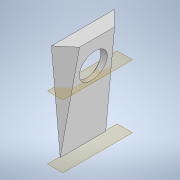
# Autodesk Inventor part: irragation01
Saved by Autodesk Inventor 2021 (Build 250183000, 183)
## iProperties
Created: 2020-07-06
Part Number: irragation01
Material: Generic
Document SubType Name: Modeling
Designer: robst
Density: 1 g/cm^3
Appearance: Default
Author: robst
Autodesk Inventor part; units mm, degrees
ref_plane "YZ Plane" through (0, 0, 0) normal (1, 0, 0) x (0, 1, 0)
ref_plane "XY Plane" through (0, 0, 0) normal (0, 0, 1) x (1, 0, 0)
sketch "Sketch1" plane through (0, 0, 0) normal (0, 0, 1) x (1, 0, 0)
  line L0 (0, 0) -> (14.2789, 101.6)
  line L1 (14.2789, 101.6) -> (0, 101.6)
  line L2 (0, 101.6) -> (0, 0)
  dimension "height" = 101.6
  dimension "d1" = 8
  dimension "d2" = 14.279
  constraints: 6 end point, 1 horizontal, 1 vertical
  measures "height" distance from line of L0.start L1
  measures "d1" angle of L0 L2
  measures "d2" distance of L0.end L1.end
extrude "MainStructure" add sketch "Sketch1" along normal mid plane 63.5
sketch "Sketch2" plane through (0, 0, 31.75) normal (-1, 0, 0) x (0, 0, 1)
  circle A0 centre (-31.75, 73.66) radius 13.97
  line L0 (-63.5, 101.6) -> (0, 101.6) projected
  line L1 (-31.75, 101.6) -> (-31.75, 0) construction
  dimension "hole" = 27.94
  dimension "centerOfHoleFromTop" = 27.94
  dimension "d29" = 0
  constraints: 2 end point, 1 centre point, 1 midpoint, 1 vertical
  measures "hole" diameter of A0
  measures "centerOfHoleFromTop" distance from line of A0.centre L0
  measures "d29" distance from line of A0.centre L1
extrude "PipeHole" cut sketch "Sketch2" against normal through all
sketch "Sketch6" plane through (0, 0, 0) normal (0, 0, 1) x (1, 0, 0)
  line L0 (0, 101.6) -> (14.2789, 101.6) projected
  line L1 (0, 0) -> (0, 101.6) projected
  line L2 (14.2789, 101.6) -> (0, 0) projected
  line L3 (0, 101.6) -> (14.1055, 100.3659)
  line L4 (14.1055, 100.3659) -> (14.2789, 101.6)
  line L5 (14.2789, 101.6) -> (0, 101.6)
  dimension "mainAngle" = 5
  constraints: 6 end point, 1 collinear, 1 point on line
  measures "mainAngle" angle of L3 L0
extrude "AngleForTopRelief" cut sketch "Sketch6" along normal through all both and the other way through all contours L0 L2 L3
sketch "Sketch7" plane through (0, 0, -31.75) normal (-1, 0, 0) x (0, 0, 1)
  line L0 (0, 0) -> (0, 101.6) construction
  line L1 (0, 44.45) -> (63.5, 44.45) construction
  line L2 (63.5, 0) -> (63.5, 100.3659) construction
  line L3 (0, 0) -> (63.5, 0) projected
  line L4 (9.9151, 38.1) -> (7.9473, 38.1)
  line L5 (7.9473, 38.1) -> (7.9473, 38.6187)
  line L6 (7.9473, 38.6187) -> (8.5936, 38.6187)
  line L7 (8.5936, 38.6187) -> (8.5936, 42.6613)
  line L8 (8.5936, 42.6613) -> (7.9473, 42.6613)
  line L9 (7.9473, 42.6613) -> (7.9473, 43.18)
  line L10 (7.9473, 43.18) -> (9.9151, 43.18)
  line L11 (9.9151, 43.18) -> (9.9151, 42.6613)
  line L12 (9.9151, 42.6613) -> (9.2687, 42.6613)
  line L13 (9.2687, 42.6613) -> (9.2687, 38.6187)
  line L14 (9.2687, 38.6187) -> (9.9151, 38.6187)
  line L15 (9.9151, 38.6187) -> (9.9151, 38.1)
  line L16 (14.6822, 38.1) -> (13.8053, 38.1)
  line L17 (13.8053, 38.1) -> (12.1998, 40.1213)
  line L18 (12.1998, 40.1213) -> (11.4259, 40.1213)
  line L19 (11.4259, 40.1213) -> (11.4259, 38.1)
  line L20 (11.4259, 38.1) -> (10.7507, 38.1)
  line L21 (10.7507, 38.1) -> (10.7507, 43.18)
  line L22 (10.7507, 43.18) -> (12.0599, 43.18)
  spline S0 degree 2 poles (12.0599, 43.18) (12.4962, 43.18) (13.0849, 43.0853) (13.3525, 42.9124) knots 0 0 0 1 2 2 2
  spline S1 degree 2 poles (13.3525, 42.9124) (13.6201, 42.7395) (13.9288, 42.2002) (13.9288, 41.8009) knots 0 0 0 1 2 2 2
  spline S2 degree 2 poles (13.9288, 41.8009) (13.9288, 41.2452) (13.3607, 40.4918) (12.875, 40.3107) knots 0 0 0 1 2 2 2
  line L23 (12.875, 40.3107) -> (14.6822, 38.1)
  spline S3 degree 2 poles (13.2249, 41.7474) (13.2249, 41.9697) (13.0684, 42.3114) (12.9038, 42.4225) knots 0 0 0 1 2 2 2
  spline S4 degree 2 poles (12.9038, 42.4225) (12.7597, 42.5172) (12.3768, 42.5954) (12.0969, 42.5954) knots 0 0 0 1 2 2 2
  line L24 (12.0969, 42.5954) -> (11.4259, 42.5954)
  line L25 (11.4259, 42.5954) -> (11.4259, 40.6853)
  line L26 (11.4259, 40.6853) -> (12.0187, 40.6853)
  spline S5 degree 2 poles (12.0187, 40.6853) (12.311, 40.6853) (12.7762, 40.7882) (12.9367, 40.9488) knots 0 0 0 1 2 2 2
  spline S6 degree 2 poles (12.9367, 40.9488) (13.0849, 41.0887) (13.2249, 41.4839) (13.2249, 41.7474) knots 0 0 0 1 2 2 2
  line L27 (19.0171, 38.1) -> (18.1402, 38.1)
  line L28 (18.1402, 38.1) -> (16.5347, 40.1213)
  line L29 (16.5347, 40.1213) -> (15.7608, 40.1213)
  line L30 (15.7608, 40.1213) -> (15.7608, 38.1)
  line L31 (15.7608, 38.1) -> (15.0856, 38.1)
  line L32 (15.0856, 38.1) -> (15.0856, 43.18)
  line L33 (15.0856, 43.18) -> (16.3947, 43.18)
  spline S7 degree 2 poles (16.3947, 43.18) (16.8311, 43.18) (17.4198, 43.0853) (17.6874, 42.9124) knots 0 0 0 1 2 2 2
  spline S8 degree 2 poles (17.6874, 42.9124) (17.955, 42.7395) (18.2637, 42.2002) (18.2637, 41.8009) knots 0 0 0 1 2 2 2
  spline S9 degree 2 poles (18.2637, 41.8009) (18.2637, 41.2452) (17.6956, 40.4918) (17.2098, 40.3107) knots 0 0 0 1 2 2 2
  line L34 (17.2098, 40.3107) -> (19.0171, 38.1)
  spline S10 degree 2 poles (17.5598, 41.7474) (17.5598, 41.9697) (17.4033, 42.3114) (17.2387, 42.4225) knots 0 0 0 1 2 2 2
  spline S11 degree 2 poles (17.2387, 42.4225) (17.0946, 42.5172) (16.7117, 42.5954) (16.4318, 42.5954) knots 0 0 0 1 2 2 2
  line L35 (16.4318, 42.5954) -> (15.7608, 42.5954)
  line L36 (15.7608, 42.5954) -> (15.7608, 40.6853)
  line L37 (15.7608, 40.6853) -> (16.3536, 40.6853)
  spline S12 degree 2 poles (16.3536, 40.6853) (16.6459, 40.6853) (17.111, 40.7882) (17.2716, 40.9488) knots 0 0 0 1 2 2 2
  spline S13 degree 2 poles (17.2716, 40.9488) (17.4198, 41.0887) (17.5598, 41.4839) (17.5598, 41.7474) knots 0 0 0 1 2 2 2
  line L38 (18.873, 38.1) -> (20.5855, 43.18)
  line L39 (20.5855, 43.18) -> (21.4171, 43.18)
  line L40 (21.4171, 43.18) -> (23.1296, 38.1)
  line L41 (23.1296, 38.1) -> (22.4175, 38.1)
  line L42 (22.4175, 38.1) -> (21.9564, 39.5203)
  line L43 (21.9564, 39.5203) -> (20.0174, 39.5203)
  line L44 (20.0174, 39.5203) -> (19.5564, 38.1)
  line L45 (19.5564, 38.1) -> (18.873, 38.1)
  line L46 (21.7711, 40.0966) -> (20.9848, 42.4884)
  line L47 (20.9848, 42.4884) -> (20.2027, 40.0966)
  line L48 (20.2027, 40.0966) -> (21.7711, 40.0966)
  spline S14 degree 2 poles (25.8055, 38.0012) (25.2662, 38.0012) (24.3729, 38.3305) (24.0518, 38.664) knots 0 0 0 1 2 2 2
  spline S15 degree 2 poles (24.0518, 38.664) (23.7307, 39.0016) (23.389, 39.9978) (23.389, 40.6441) knots 0 0 0 1 2 2 2
  spline S16 degree 2 poles (23.389, 40.6441) (23.389, 41.2575) (23.7348, 42.229) (24.0559, 42.5748) knots 0 0 0 1 2 2 2
  spline S17 degree 2 poles (24.0559, 42.5748) (24.3647, 42.9083) (25.2703, 43.2706) (25.8096, 43.2706) knots 0 0 0 1 2 2 2
  spline S18 degree 2 poles (25.8096, 43.2706) (26.069, 43.2706) (26.5383, 43.1965) (26.7523, 43.1306) knots 0 0 0 1 2 2 2
  spline S19 degree 2 poles (26.7523, 43.1306) (26.9252, 43.0812) (27.3451, 42.9001) (27.4728, 42.8342) knots 0 0 0 1 2 2 2
  line L49 (27.4728, 42.8342) -> (27.4728, 42.0191)
  line L50 (27.4728, 42.0191) -> (27.4151, 42.0191)
  spline S20 degree 2 poles (27.4151, 42.0191) (27.2875, 42.1302) (27.0199, 42.332) (26.7729, 42.4472) knots 0 0 0 1 2 2 2
  spline S21 degree 2 poles (26.7729, 42.4472) (26.5671, 42.5501) (26.036, 42.686) (25.7314, 42.686) knots 0 0 0 1 2 2 2
  spline S22 degree 2 poles (25.7314, 42.686) (24.9986, 42.686) (24.0929, 41.5827) (24.0929, 40.6647) knots 0 0 0 1 2 2 2
  spline S23 degree 2 poles (24.0929, 40.6647) (24.0929, 40.1542) (24.3317, 39.3885) (24.5581, 39.1251) knots 0 0 0 1 2 2 2
  spline S24 degree 2 poles (24.5581, 39.1251) (24.7763, 38.8616) (25.3938, 38.5858) (25.7808, 38.5858) knots 0 0 0 1 2 2 2
  spline S25 degree 2 poles (25.7808, 38.5858) (26.0648, 38.5858) (26.6329, 38.6681) (26.8264, 38.7504) knots 0 0 0 1 2 2 2
  line L51 (26.8264, 38.7504) -> (26.8264, 40.0637)
  line L52 (26.8264, 40.0637) -> (25.6491, 40.0637)
  line L53 (25.6491, 40.0637) -> (25.6491, 40.6565)
  line L54 (25.6491, 40.6565) -> (27.4933, 40.6565)
  line L55 (27.4933, 40.6565) -> (27.4933, 38.4376)
  spline S26 degree 2 poles (27.4933, 38.4376) (27.3657, 38.3799) (26.9294, 38.2029) (26.7441, 38.1494) knots 0 0 0 1 2 2 2
  spline S27 degree 2 poles (26.7441, 38.1494) (26.493, 38.0753) (26.0895, 38.0012) (25.8055, 38.0012) knots 0 0 0 1 2 2 2
  line L56 (27.7939, 38.1) -> (29.5064, 43.18)
  line L57 (29.5064, 43.18) -> (30.338, 43.18)
  line L58 (30.338, 43.18) -> (32.0505, 38.1)
  line L59 (32.0505, 38.1) -> (31.3383, 38.1)
  line L60 (31.3383, 38.1) -> (30.8773, 39.5203)
  line L61 (30.8773, 39.5203) -> (28.9383, 39.5203)
  line L62 (28.9383, 39.5203) -> (28.4772, 38.1)
  line L63 (28.4772, 38.1) -> (27.7939, 38.1)
  line L64 (30.692, 40.0966) -> (29.9057, 42.4884)
  line L65 (29.9057, 42.4884) -> (29.1235, 40.0966)
  line L66 (29.1235, 40.0966) -> (30.692, 40.0966)
  line L67 (33.7836, 38.1) -> (33.7836, 42.579)
  line L68 (33.7836, 42.579) -> (32.0793, 42.579)
  line L69 (32.0793, 42.579) -> (32.0793, 43.18)
  line L70 (32.0793, 43.18) -> (36.1631, 43.18)
  line L71 (36.1631, 43.18) -> (36.1631, 42.579)
  line L72 (36.1631, 42.579) -> (34.4588, 42.579)
  line L73 (34.4588, 42.579) -> (34.4588, 38.1)
  line L74 (34.4588, 38.1) -> (33.7836, 38.1)
  line L75 (38.452, 38.1) -> (36.4842, 38.1)
  line L76 (36.4842, 38.1) -> (36.4842, 38.6187)
  line L77 (36.4842, 38.6187) -> (37.1305, 38.6187)
  line L78 (37.1305, 38.6187) -> (37.1305, 42.6613)
  line L79 (37.1305, 42.6613) -> (36.4842, 42.6613)
  line L80 (36.4842, 42.6613) -> (36.4842, 43.18)
  line L81 (36.4842, 43.18) -> (38.452, 43.18)
  line L82 (38.452, 43.18) -> (38.452, 42.6613)
  line L83 (38.452, 42.6613) -> (37.8057, 42.6613)
  line L84 (37.8057, 42.6613) -> (37.8057, 38.6187)
  line L85 (37.8057, 38.6187) -> (38.452, 38.6187)
  line L86 (38.452, 38.6187) -> (38.452, 38.1)
  spline S28 degree 2 poles (42.8815, 42.5995) (43.1697, 42.262) (43.4908, 41.274) (43.4908, 40.64) knots 0 0 0 1 2 2 2
  spline S29 degree 2 poles (43.4908, 40.64) (43.4908, 40.0225) (43.1779, 39.0221) (42.8815, 38.6846) knots 0 0 0 1 2 2 2
  spline S30 degree 2 poles (42.8815, 38.6846) (42.5687, 38.3305) (41.7412, 37.993) (41.2431, 37.993) knots 0 0 0 1 2 2 2
  spline S31 degree 2 poles (41.2431, 37.993) (40.7285, 37.993) (39.9052, 38.3429) (39.6047, 38.6846) knots 0 0 0 1 2 2 2
  spline S32 degree 2 poles (39.6047, 38.6846) (39.3124, 39.0221) (38.9995, 40.0143) (38.9995, 40.64) knots 0 0 0 1 2 2 2
  spline S33 degree 2 poles (38.9995, 40.64) (38.9995, 41.2781) (39.3165, 42.2496) (39.6088, 42.5995) knots 0 0 0 1 2 2 2
  spline S34 degree 2 poles (39.6088, 42.5995) (39.9052, 42.9371) (40.7326, 43.287) (41.2431, 43.287) knots 0 0 0 1 2 2 2
  spline S35 degree 2 poles (41.2431, 43.287) (41.7618, 43.287) (42.5934, 42.9248) (42.8815, 42.5995) knots 0 0 0 1 2 2 2
  spline S36 degree 2 poles (42.7869, 40.64) (42.7869, 41.1422) (42.5687, 41.9203) (42.3711, 42.1755) knots 0 0 0 1 2 2 2
  spline S37 degree 2 poles (42.3711, 42.1755) (42.1694, 42.439) (41.6012, 42.7025) (41.2472, 42.7025) knots 0 0 0 1 2 2 2
  spline S38 degree 2 poles (41.2472, 42.7025) (40.8808, 42.7025) (40.3292, 42.4472) (40.1192, 42.1755) knots 0 0 0 1 2 2 2
  spline S39 degree 2 poles (40.1192, 42.1755) (39.9175, 41.9162) (39.7035, 41.134) (39.7035, 40.64) knots 0 0 0 1 2 2 2
  spline S40 degree 2 poles (39.7035, 40.64) (39.7035, 39.6396) (40.5433, 38.5775) (41.2472, 38.5775) knots 0 0 0 1 2 2 2
  spline S41 degree 2 poles (41.2472, 38.5775) (41.9512, 38.5775) (42.7869, 39.6396) (42.7869, 40.64) knots 0 0 0 1 2 2 2
  line L87 (47.8669, 38.1) -> (47.1094, 38.1)
  line L88 (47.1094, 38.1) -> (44.8617, 42.4802)
  line L89 (44.8617, 42.4802) -> (44.8617, 38.1)
  line L90 (44.8617, 38.1) -> (44.2318, 38.1)
  line L91 (44.2318, 38.1) -> (44.2318, 43.18)
  line L92 (44.2318, 43.18) -> (45.191, 43.18)
  line L93 (45.191, 43.18) -> (47.237, 39.158)
  line L94 (47.237, 39.158) -> (47.237, 43.18)
  line L95 (47.237, 43.18) -> (47.8669, 43.18)
  line L96 (47.8669, 43.18) -> (47.8669, 38.1)
  spline S42 degree 2 poles (51.9136, 40.64) (51.9136, 39.2733) (51.119, 37.993) (50.2916, 37.993) knots 0 0 0 1 2 2 2
  spline S43 degree 2 poles (50.2916, 37.993) (49.4518, 37.993) (48.6655, 39.298) (48.6655, 40.6359) knots 0 0 0 1 2 2 2
  spline S44 degree 2 poles (48.6655, 40.6359) (48.6655, 42.0109) (49.46, 43.2829) (50.2916, 43.2829) knots 0 0 0 1 2 2 2
  spline S45 degree 2 poles (50.2916, 43.2829) (51.1273, 43.2829) (51.9136, 41.9656) (51.9136, 40.64) knots 0 0 0 1 2 2 2
  spline S46 degree 2 poles (51.0408, 39.0921) (51.1396, 39.3432) (51.222, 40.1172) (51.222, 40.64) knots 0 0 0 1 2 2 2
  spline S47 degree 2 poles (51.222, 40.64) (51.222, 41.1628) (51.1396, 41.9326) (51.0367, 42.192) knots 0 0 0 1 2 2 2
  spline S48 degree 2 poles (51.0367, 42.192) (50.9338, 42.4513) (50.5756, 42.7189) (50.2916, 42.7189) knots 0 0 0 1 2 2 2
  spline S49 degree 2 poles (50.2916, 42.7189) (50.0075, 42.7189) (49.6412, 42.4513) (49.5341, 42.1838) knots 0 0 0 1 2 2 2
  spline S50 degree 2 poles (49.5341, 42.1838) (49.4312, 41.9244) (49.3571, 41.134) (49.3571, 40.6359) knots 0 0 0 1 2 2 2
  spline S51 degree 2 poles (49.3571, 40.6359) (49.3571, 40.1007) (49.423, 39.3844) (49.53, 39.1045) knots 0 0 0 1 2 2 2
  spline S52 degree 2 poles (49.53, 39.1045) (49.6288, 38.841) (49.9952, 38.557) (50.2916, 38.557) knots 0 0 0 1 2 2 2
  spline S53 degree 2 poles (50.2916, 38.557) (50.5715, 38.557) (50.9379, 38.8245) (51.0408, 39.0921) knots 0 0 0 1 2 2 2
  line L97 (55.4416, 38.1) -> (52.9633, 38.1)
  line L98 (52.9633, 38.1) -> (52.9633, 38.6187)
  line L99 (52.9633, 38.6187) -> (53.8855, 38.6187)
  line L100 (53.8855, 38.6187) -> (53.8855, 42.0232)
  line L101 (53.8855, 42.0232) -> (52.9633, 42.0232)
  line L102 (52.9633, 42.0232) -> (52.9633, 42.4884)
  spline S54 degree 2 poles (52.9633, 42.4884) (53.4861, 42.4884) (53.9801, 42.7848) (54.0131, 43.1965) knots 0 0 0 1 2 2 2
  line L103 (54.0131, 43.1965) -> (54.54, 43.1965)
  line L104 (54.54, 43.1965) -> (54.54, 38.6187)
  line L105 (54.54, 38.6187) -> (55.4416, 38.6187)
  line L106 (55.4416, 38.6187) -> (55.4416, 38.1)
  point P0 (31.75, 0)
  dimension "lineForText" = 44.45
  constraints: 2 end point, 2 horizontal, 2 point on line
  measures "lineForText" distance between parallel lines of L3 L1
extrude "TextForBack" cut sketch "Sketch7" against normal blind 1.905
sketch "Sketch8" plane through (0, 0, -31.75) normal (-1, 0, 0) x (0, 0, 1)
  circle A0 centre (31.75, 73.66) radius 13.97 projected
  circle A1 centre (31.75, 73.66) radius 19.05
  point P0 (31.75, 0)
  dimension "reliefHoleDiameter" = 38.1
  constraints: 1 centre point, 1 coincident
  measures "reliefHoleDiameter" diameter of A1
extrude "ReliefForHole" cut sketch "Sketch8" against normal blind 3.81 contours A0 | A1
sketch "Sketch9" plane through (0, 0, -31.75) normal (-1, 0, 0) x (0, 0, 1)
  line L0 (0, 100.3659) -> (0, 0) projected
  line L1 (0, 92.075) -> (63.5, 92.075) construction
  line L2 (63.5, 0) -> (63.5, 100.3659) projected
  line L3 (0, 101.6) -> (63.5, 101.6) construction
  spline S0 degree 2 poles (17.4664, 90.2379) (17.4664, 89.5278) (16.926, 88.4394) (16.4784, 88.0844) knots 0 0 0 1 2 2 2
  spline S1 degree 2 poles (16.4784, 88.0844) (15.938, 87.6676) (14.7107, 87.3125) (13.7382, 87.3125) knots 0 0 0 1 2 2 2
  line L4 (13.7382, 87.3125) -> (11.0057, 87.3125)
  line L5 (11.0057, 87.3125) -> (11.0057, 96.8375)
  line L6 (11.0057, 96.8375) -> (13.5298, 96.8375)
  spline S2 degree 2 poles (13.5298, 96.8375) (14.5487, 96.8375) (15.5675, 96.7063) (16.0307, 96.4516) knots 0 0 0 1 2 2 2
  spline S3 degree 2 poles (16.0307, 96.4516) (16.5478, 96.1814) (17.0187, 95.2937) (17.0187, 94.6917) knots 0 0 0 1 2 2 2
  spline S4 degree 2 poles (17.0187, 94.6917) (17.0187, 94.0201) (16.3085, 92.9549) (15.6833, 92.6539) knots 0 0 0 1 2 2 2
  line L7 (15.6833, 92.6539) -> (15.6833, 92.6076)
  spline S5 degree 2 poles (15.6833, 92.6076) (16.5324, 92.376) (17.4664, 91.1487) (17.4664, 90.2379) knots 0 0 0 1 2 2 2
  spline S6 degree 2 poles (16.1464, 90.1839) (16.1464, 90.7242) (15.8377, 91.4189) (15.3746, 91.6659) knots 0 0 0 1 2 2 2
  spline S7 degree 2 poles (15.3746, 91.6659) (15.0735, 91.8203) (14.3634, 91.9129) (13.7073, 91.9129) knots 0 0 0 1 2 2 2
  line L8 (13.7073, 91.9129) -> (12.2716, 91.9129)
  line L9 (12.2716, 91.9129) -> (12.2716, 88.3931)
  line L10 (12.2716, 88.3931) -> (13.2982, 88.3931)
  spline S8 degree 2 poles (13.2982, 88.3931) (14.1318, 88.3931) (15.089, 88.5475) (15.4595, 88.7945) knots 0 0 0 1 2 2 2
  spline S9 degree 2 poles (15.4595, 88.7945) (15.8145, 89.0492) (16.1464, 89.6822) (16.1464, 90.1839) knots 0 0 0 1 2 2 2
  spline S10 degree 2 poles (15.6988, 94.5141) (15.6988, 94.8538) (15.4672, 95.3632) (15.2125, 95.5099) knots 0 0 0 1 2 2 2
  spline S11 degree 2 poles (15.2125, 95.5099) (14.9037, 95.6797) (14.155, 95.7569) (13.4835, 95.7569) knots 0 0 0 1 2 2 2
  line L11 (13.4835, 95.7569) -> (12.2716, 95.7569)
  line L12 (12.2716, 95.7569) -> (12.2716, 92.9704)
  line L13 (12.2716, 92.9704) -> (13.7073, 92.9704)
  spline S12 degree 2 poles (13.7073, 92.9704) (14.3017, 92.9704) (14.8651, 93.0939) (15.1662, 93.2869) knots 0 0 0 1 2 2 2
  spline S13 degree 2 poles (15.1662, 93.2869) (15.4595, 93.4721) (15.6988, 94.0665) (15.6988, 94.5141) knots 0 0 0 1 2 2 2
  line L14 (21.7889, 87.3125) -> (24.9999, 96.8375)
  line L15 (24.9999, 96.8375) -> (26.5591, 96.8375)
  line L16 (26.5591, 96.8375) -> (29.7701, 87.3125)
  line L17 (29.7701, 87.3125) -> (28.4348, 87.3125)
  line L18 (28.4348, 87.3125) -> (27.5703, 89.9755)
  line L19 (27.5703, 89.9755) -> (23.9347, 89.9755)
  line L20 (23.9347, 89.9755) -> (23.0702, 87.3125)
  line L21 (23.0702, 87.3125) -> (21.7889, 87.3125)
  line L22 (27.2229, 91.0561) -> (25.7486, 95.5407)
  line L23 (25.7486, 95.5407) -> (24.2821, 91.0561)
  line L24 (24.2821, 91.0561) -> (27.2229, 91.0561)
  spline S14 degree 2 poles (38.6082, 87.1427) (37.6819, 87.1427) (36.115, 87.7679) (35.5438, 88.3931) knots 0 0 0 1 2 2 2
  spline S15 degree 2 poles (35.5438, 88.3931) (34.9726, 89.0106) (34.3474, 90.8631) (34.3474, 92.0673) knots 0 0 0 1 2 2 2
  spline S16 degree 2 poles (34.3474, 92.0673) (34.3474, 93.2637) (34.9572, 95.039) (35.5361, 95.6951) knots 0 0 0 1 2 2 2
  spline S17 degree 2 poles (35.5361, 95.6951) (36.1073, 96.3358) (37.6665, 97.0073) (38.6313, 97.0073) knots 0 0 0 1 2 2 2
  spline S18 degree 2 poles (38.6313, 97.0073) (39.1099, 97.0073) (39.9512, 96.8684) (40.3063, 96.7603) knots 0 0 0 1 2 2 2
  spline S19 degree 2 poles (40.3063, 96.7603) (40.615, 96.66) (41.2557, 96.3744) (41.5722, 96.2046) knots 0 0 0 1 2 2 2
  line L25 (41.5722, 96.2046) -> (41.5722, 94.6762)
  line L26 (41.5722, 94.6762) -> (41.4718, 94.6762)
  spline S20 degree 2 poles (41.4718, 94.6762) (41.302, 94.8306) (40.7771, 95.2629) (40.3989, 95.4713) knots 0 0 0 1 2 2 2
  spline S21 degree 2 poles (40.3989, 95.4713) (40.0361, 95.672) (39.1793, 95.9267) (38.6236, 95.9267) knots 0 0 0 1 2 2 2
  spline S22 degree 2 poles (38.6236, 95.9267) (38.0138, 95.9267) (36.9255, 95.425) (36.5164, 94.9464) knots 0 0 0 1 2 2 2
  spline S23 degree 2 poles (36.5164, 94.9464) (36.115, 94.4601) (35.6673, 92.9858) (35.6673, 92.0673) knots 0 0 0 1 2 2 2
  spline S24 degree 2 poles (35.6673, 92.0673) (35.6673, 91.087) (36.1381, 89.6745) (36.5472, 89.1882) knots 0 0 0 1 2 2 2
  spline S25 degree 2 poles (36.5472, 89.1882) (36.9486, 88.7173) (38.0215, 88.2388) (38.6236, 88.2388) knots 0 0 0 1 2 2 2
  spline S26 degree 2 poles (38.6236, 88.2388) (39.1716, 88.2388) (40.1056, 88.5089) (40.4684, 88.7096) knots 0 0 0 1 2 2 2
  spline S27 degree 2 poles (40.4684, 88.7096) (40.8157, 88.9103) (41.3329, 89.3271) (41.4795, 89.4738) knots 0 0 0 1 2 2 2
  line L27 (41.4795, 89.4738) -> (41.5722, 89.4738)
  line L28 (41.5722, 89.4738) -> (41.5722, 87.9609)
  spline S28 degree 2 poles (41.5722, 87.9609) (41.2557, 87.8142) (40.7, 87.5441) (40.3063, 87.4206) knots 0 0 0 1 2 2 2
  spline S29 degree 2 poles (40.3063, 87.4206) (39.8895, 87.2816) (39.1793, 87.1427) (38.6082, 87.1427) knots 0 0 0 1 2 2 2
  line L29 (53.791, 87.3125) -> (52.1469, 87.3125)
  line L30 (52.1469, 87.3125) -> (48.6658, 91.7431)
  line L31 (48.6658, 91.7431) -> (48.11, 91.1179)
  line L32 (48.11, 91.1179) -> (48.11, 87.3125)
  line L33 (48.11, 87.3125) -> (46.8441, 87.3125)
  line L34 (46.8441, 87.3125) -> (46.8441, 96.8375)
  line L35 (46.8441, 96.8375) -> (48.11, 96.8375)
  line L36 (48.11, 96.8375) -> (48.11, 92.4609)
  line L37 (48.11, 92.4609) -> (52.0157, 96.8375)
  line L38 (52.0157, 96.8375) -> (53.5595, 96.8375)
  line L39 (53.5595, 96.8375) -> (49.6152, 92.5844)
  line L40 (49.6152, 92.5844) -> (53.791, 87.3125)
  point P0 (31.75, 0)
  dimension "d35" = 9.525
  constraints: 2 end point, 2 horizontal, 2 point on line
  measures "d35" distance between parallel lines of L1 L3
extrude "TextForSmallText" cut sketch "Sketch9" against normal blind 2.54
ref_plane "Work Plane1" through (0, 101.6, 31.75) normal (0, 1, 0) x (-1, 0, 0)
sketch "Sketch10" plane through (14.1055, 100.3659, 31.75) normal (0.0871557, 0.9961947, 0) x (0.9961947, -0.0871557, 0)
  line L0 (-14.1594, 63.5) -> (-14.1594, 0) projected
  line L1 (0, 0) -> (-14.1594, 0) projected
  line L2 (0, 63.5) -> (0, 0) projected
  line L3 (-14.1594, 0) -> (0, 14.1594)
  line L4 (-14.1594, 0) -> (5.865, 0) construction
  line L5 (0, 14.1594) -> (0, 0)
  line L6 (0, 0) -> (-14.1594, 0)
  line L7 (-14.1594, 63.5) -> (0, 63.5) projected
  line L8 (-14.1594, 63.5) -> (0, 49.3406)
  line L9 (-14.1594, 63.5) -> (5.865, 63.5) construction
  line L10 (0, 49.3406) -> (0, 63.5)
  line L11 (0, 63.5) -> (-14.1594, 63.5)
  point P0 (-5.3044, 31.75)
  dimension "d38" = 45
  dimension "d39" = 45
  constraints: 16 end point, 2 collinear, 2 equal length, 2 horizontal, 2 point on line
  measures "d38" angle of L4 L3
  measures "d39" angle of L8 L9
extrude "SideAngle" cut sketch "Sketch10" against normal through all contours L7 L2 L8 | L3 L2 L1
ref_plane "Work Plane2" through (0, 63.5, 0) normal (0, 1, 0) x (-1, 0, 0)
body "Solid1"
